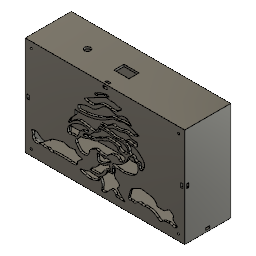
Classroom quality sensor (Autodesk Fusion 360 design; units mm, degrees)
Autodesk Fusion 360 part; units mm, degrees
(part 1 of 2)
sketch "Box (main and holes)" plane through (0, 0, 0) normal (0, 0, 1) x (1, 0, 0)
  line L0 (77.5, 47.5) -> (-77.5, 47.5)
  line L1 (-77.5, 47.5) -> (-77.5, -47.5)
  line L2 (-77.5, -47.5) -> (77.5, -47.5)
  line L3 (77.5, -47.5) -> (77.5, 47.5)
  line L4 (77.5, 47.5) -> (-77.5, -47.5) construction
  line L5 (-77.5, 47.5) -> (77.5, -47.5) construction
  line L6 (-79.5, 49.5) -> (79.5, 49.5)
  line L7 (79.5, 49.5) -> (79.5, -49.5)
  line L8 (79.5, -49.5) -> (-79.5, -49.5)
  line L9 (-79.5, -49.5) -> (-79.5, 49.5)
  line L10 (-79.5, 49.5) -> (79.5, -49.5) construction
  line L11 (79.5, 49.5) -> (-79.5, -49.5) construction
  line L12 (-77.5, -47.5) -> (-77.5, -49.5)
  line L13 (77.5, -47.5) -> (77.5, -49.5)
  dimension "d5" = 155
  dimension "d6" = 95
  dimension "d7" = 2
  dimension "d8" = 2
  constraint horizontal L0
  constraint perpendicular L0 L1
  constraint parallel L0 L2
  constraint parallel L1 L3
  constraint coincident L4 origin
  constraint coincident L5 origin
  constraint horizontal L6
  constraint perpendicular L6 L7
  constraint parallel L6 L8
  constraint parallel L7 L9
  constraint coincident L10 origin
  constraint coincident L11 origin
  constraint coincident L8 L12.end
  constraint perpendicular L8 L12
  constraint coincident L8 L13.end
  constraint perpendicular L8 L13
  measures "d5" distance of L1.end L2.end
  measures "d6" distance of L0.end L1.end
  measures "d7" distance of L2 L8
  measures "d8" distance of L1 L9
extrude "Extrude1" add sketch "Box (main and holes)" against normal blind 2 makes body 1
extrude "Extrude2" add sketch "Box (main and holes)" along normal blind 44 contours L0 L1 L3 L6 L7 L8 L9 L12 L13 bodies 1
chamfer "Chamfer2" distance 2 angle 45 6 edges at (0, -49.5, 0) (-77.5, -49.5, 22) (-77.5, -1, 44) (77.5, -49.5, 22) (77.5, -1, 44) (0, 47.5, 44) on bodies 1
sketch "Box (guides and top holes)" plane through (0, 47.5, 0) normal (0, -1, 0) x (1, 0, 0)
  line L0 (77.5, 42) -> (-77.5, 42)
  line L1 (-77.5, 42) -> (-77.5, 0)
  line L2 (-77.5, 0) -> (77.5, 0)
  line L3 (77.5, 0) -> (77.5, 42)
  line L4 (-77.5, 5) -> (-72.5, 5)
  line L5 (-72.5, 5) -> (-72.5, 7)
  line L6 (-72.5, 7) -> (-77.5, 7)
  line L7 (-77.5, 7) -> (-77.5, 5)
  line L8 (-77.5, 10) -> (-72.5, 10)
  line L9 (-72.5, 10) -> (-72.5, 12)
  line L10 (-72.5, 12) -> (-77.5, 12)
  line L11 (-77.5, 12) -> (-77.5, 10)
  line L12 (-77.5, 42) -> (77.5, 42) construction
  line L13 (72.5, 12) -> (77.5, 12)
  line L14 (77.5, 12) -> (77.5, 10)
  line L15 (77.5, 10) -> (72.5, 10)
  line L16 (72.5, 10) -> (72.5, 12)
  line L17 (72.5, 7) -> (77.5, 7)
  line L18 (77.5, 7) -> (77.5, 5)
  line L19 (77.5, 5) -> (72.5, 5)
  line L20 (72.5, 5) -> (72.5, 7)
  line L21 (0, 1.75) -> (0, 22.5)
  line L22 (2, 42) -> (-2, 42)
  line L23 (-2, 42) -> (-2, 40)
  line L24 (-2, 40) -> (2, 40)
  line L25 (2, 40) -> (2, 42)
  line L26 (2, 42) -> (-2, 40) construction
  line L27 (-2, 42) -> (2, 40) construction
  line L28 (-77.5, 10) -> (77.5, 10) construction
  line L29 (0, 10) -> (0, 22.5) construction
  line L30 (7.5, 27.5) -> (-7.5, 27.5)
  line L31 (-7.5, 27.5) -> (-7.5, 17.5)
  line L32 (-7.5, 17.5) -> (7.5, 17.5)
  line L33 (7.5, 17.5) -> (7.5, 27.5)
  line L34 (7.5, 27.5) -> (-7.5, 17.5) construction
  line L35 (-7.5, 27.5) -> (7.5, 17.5) construction
  line L36 (-38.75, 10) -> (-38.75, 22.5) construction
  circle A0 centre (-38.75, 22.5) radius 3
  point P0 (0, 41)
  point P1 (0, 42)
  point P2 (0, 42)
  point P3 (0, 22.5)
  dimension "d15" = 5
  dimension "d16" = 2
  dimension "d23" = 5
  dimension "d26" = 3
  dimension "d27" = 30
  dimension "d31" = 4
  dimension "d32" = 2
  dimension "d51" = 12.5
  dimension "d52" = 15
  dimension "d53" = 10
  dimension "d54" = 12.5
  dimension "d55" = 38.75
  dimension "d56" = 6
  constraint horizontal L4
  constraint vertical L5
  constraint horizontal L6
  constraint vertical L7
  constraint coincident L1 L4.start
  constraint horizontal L8
  constraint vertical L9
  constraint horizontal L10
  constraint vertical L11
  constraint coincident L1 L8.start
  constraint coincident L1 L0.end
  constraint coincident L3 L0.start
  constraint perpendicular L3 L12
  constraint equal L6 L10
  constraint equal L5 L9
  constraint horizontal L13
  constraint vertical L14
  constraint horizontal L15
  constraint vertical L16
  constraint horizontal L17
  constraint vertical L18
  constraint horizontal L19
  constraint vertical L20
  constraint symmetric L9 L16 L21
  constraint symmetric L8 L15 L21
  constraint symmetric L10 L13 L21
  constraint symmetric L11 L14 L21
  constraint symmetric L4 L19 L21
  constraint symmetric L6 L17 L21
  constraint symmetric L7 L18 L21
  constraint symmetric L5 L20 L21
  constraint horizontal L22
  constraint perpendicular L22 L23
  constraint parallel L22 L24
  constraint parallel L23 L25
  constraint coincident L26 P0
  constraint coincident L27 P0
  constraint midpoint L22 P2
  constraint midpoint L0 P2
  constraint coincident P2 P1
  constraint perpendicular L11 L28
  constraint perpendicular L28 L29
  constraint horizontal L30
  constraint perpendicular L30 L31
  constraint parallel L30 L32
  constraint parallel L31 L33
  constraint coincident L34 P3
  constraint coincident L35 P3
  constraint coincident P3 L21.end
  constraint midpoint L28 L29.start
  constraint coincident L14.end L15.start
  constraint coincident L28 L36.start
  constraint perpendicular L28 L36
  constraint coincident L36.end A0.centre
  measures "d15" distance of L4.start L4.end
  measures "d16" distance of L4.start L6.end
  measures "d23" distance of L2 L4
  measures "d26" distance of L6 L8
  measures "d27" distance of L10 L12
  measures "d31" distance of L23.end L24.end
  measures "d32" distance of L22.end L23.end
  measures "d51" distance of L29.start P3
  measures "d52" distance of L31.end L32.end
  measures "d53" distance of L30.end L31.end
  measures "d54" distance of L36.start L36.end
  measures "d55" distance of L29 L36
  measures "d56" diameter of A0
extrude "Extrude8" cut sketch "Box (guides and top holes)" against normal up to surface (2 mm away) contours L30 L31 L32 L33 | A0 bodies 1
extrude "Extrude3" add sketch "Box (guides and top holes)" along normal blind 95 contours L3 L13 L14 L15 L16 | L3 L17 L18 L19 L20 | L1 L8 L9 L10 L11 | L1 L4 L5 L6 L7 bodies 1
extrude "Extrude4" cut sketch "Box (guides and top holes)" against normal up to surface (2 mm away) contours L0 L22 L23 L24 L25 bodies 1
sketch "Box (back hole)" plane through (0, 0, -2) normal (0, 0, -1) x (-1, 0, 0)
  line L0 (-79.5, -49.5) -> (79.5, -49.5)
  line L1 (79.5, -49.5) -> (79.5, 49.5)
  line L2 (79.5, 49.5) -> (-79.5, 49.5)
  line L3 (-79.5, 49.5) -> (-79.5, -49.5)
  line L4 (2, -45.5) -> (-2, -45.5)
  line L5 (-2, -45.5) -> (-2, -47.5)
  line L6 (-2, -47.5) -> (2, -47.5)
  line L7 (2, -47.5) -> (2, -45.5)
  line L8 (2, -45.5) -> (-2, -47.5) construction
  line L9 (-2, -45.5) -> (2, -47.5) construction
  line L10 (0, -49.5) -> (0, -47.5) construction
  point P0 (0, -46.5)
  point P1 (0, -47.5)
  dimension "d36" = 4
  dimension "d37" = 2
  dimension "d48" = 2
  constraint horizontal L4
  constraint perpendicular L4 L5
  constraint parallel L4 L6
  constraint parallel L5 L7
  constraint coincident L8 P0
  constraint coincident L9 P0
  constraint midpoint L6 P1
  constraint midpoint L0 L10.start
  constraint perpendicular L0 L10
  constraint coincident P1 L10.end
  measures "d36" distance of L5.end L6.end
  measures "d37" distance of L4.end L5.end
  measures "d48" distance of L10.start P1
extrude "Extrude7" cut sketch "Box (back hole)" against normal up to surface (2 mm away) contours L4 L5 L6 L7 bodies 1
extrude "Extrude5" cut sketch "Box (back hole)" against normal up to surface (2 mm away) contours L4 L5 L6 L7 bodies 1
sketch "Box (side holes)" plane through (79.5, 0, 0) normal (1, 0, 0) x (0, 0, -1)
  line L0 (-44, -49.5) -> (2, -49.5)
  line L1 (2, -49.5) -> (2, 49.5)
  line L2 (2, 49.5) -> (-44, 49.5)
  line L3 (-44, 49.5) -> (-44, -49.5)
  line L4 (-21, -49.5) -> (-21, -47.5) construction
  line L5 (-44, 0) -> (-42, 0) construction
  line L6 (-42, 2) -> (-40, 2)
  line L7 (-40, 2) -> (-40, -2)
  line L8 (-40, -2) -> (-42, -2)
  line L9 (-42, -2) -> (-42, 2)
  line L10 (-42, 2) -> (-40, -2) construction
  line L11 (-40, 2) -> (-42, -2) construction
  line L12 (-19, -45.5) -> (-23, -45.5)
  line L13 (-23, -45.5) -> (-23, -47.5)
  line L14 (-23, -47.5) -> (-19, -47.5)
  line L15 (-19, -47.5) -> (-19, -45.5)
  line L16 (-19, -45.5) -> (-23, -47.5) construction
  line L17 (-23, -45.5) -> (-19, -47.5) construction
  point P0 (-41, 0)
  point P1 (-21, -46.5)
  point P2 (-42, 0)
  point P3 (-21, -47.5)
  dimension "d40" = 2
  dimension "d41" = 2
  dimension "d42" = 2
  dimension "d43" = 4
  dimension "d44" = 4
  dimension "d45" = 2
  constraint midpoint L0 L4.start
  constraint vertical L4
  constraint midpoint L3 L5.start
  constraint horizontal L5
  constraint horizontal L6
  constraint perpendicular L6 L7
  constraint parallel L6 L8
  constraint parallel L7 L9
  constraint coincident L10 P0
  constraint coincident L11 P0
  constraint horizontal L12
  constraint perpendicular L12 L13
  constraint parallel L12 L14
  constraint parallel L13 L15
  constraint coincident L16 P1
  constraint coincident L17 P1
  constraint midpoint L9 P2
  constraint coincident L5 P2
  constraint coincident P2 L5.end
  constraint midpoint L14 P3
  constraint coincident L4 P3
  constraint coincident P3 L4.end
  measures "d40" distance of L4.start P3
  measures "d41" distance of L5.start P2
  measures "d42" distance of L7.end L8.end
  measures "d43" distance of L6.end L7.end
  measures "d44" distance of L13.end L14.end
  measures "d45" distance of L12.end L13.end
extrude "Extrude6" cut sketch "Box (side holes)" against normal up to surface (159 mm away) contours L6 L7 L8 L9 | L12 L13 L14 L15 bodies 1
ref_plane "WorkPlane4" through (77.5, -2, 42) normal (0, 0, 1) x (1, 0, 0)
sketch "Lid (main and holes)" plane through (77.5, -2, 42) normal (0, 0, 1) x (1, 0, 0)
  line L0 (0, 49.5) -> (-155, 49.5) construction
  line L1 (-155, 49.5) -> (-155, -45.5) construction
  line L2 (-155, -45.5) -> (0, -45.5)
  line L3 (0, -45.5) -> (0, 49.5) construction
  line L4 (0, -45.5) -> (-155, 49.5) construction
  line L5 (0, 49.5) -> (-155, -45.5) construction
  line L6 (2, 51.5) -> (-157, 51.5)
  line L7 (-157, 51.5) -> (-157, -47.5)
  line L8 (-157, -47.5) -> (2, -47.5)
  line L9 (2, -47.5) -> (2, 51.5)
  line L10 (2, 51.5) -> (-157, -47.5) construction
  line L11 (-157, 51.5) -> (2, -47.5) construction
  line L12 (-155, -45.5) -> (-157, -45.5)
  line L13 (0, -45.5) -> (2, -45.5)
  spline S0 degree 3 poles (-80.6772, -42.0006) (-80.6772, -41.7695) (-80.5006, -40.5665) (-80.2848, -39.3272) knots 0 0 0 0 1 1 1 1
  spline S1 degree 3 poles (-80.2848, -39.3272) (-79.814, -36.6234) (-80.4696, -33.7851) (-81.9287, -32.2107) knots 0 0 0 0 1 1 1 1
  spline S2 degree 3 poles (-81.9287, -32.2107) (-82.4275, -31.6725) (-82.8356, -31.1623) (-82.8356, -31.0769) knots 0 0 0 0 1 1 1 1
  spline S3 degree 3 poles (-82.8356, -31.0769) (-82.8356, -30.9915) (-82.0667, -30.5302) (-81.1269, -30.0518) knots 0 0 0 0 1 1 1 1
  spline S4 degree 3 poles (-81.1269, -30.0518) (-79.0239, -28.9814) (-78.0158, -27.9242) (-76.3554, -25.048) knots 0 0 0 0 1 1 1 1
  line L14 (-76.3554, -25.048) -> (-75.0666, -22.8156)
  line L15 (-75.0666, -22.8156) -> (-72.386, -22.6357)
  line L16 (-72.386, -22.6357) -> (-69.7055, -22.4559)
  line L17 (-69.7055, -22.4559) -> (-69.7714, -21.3767)
  spline S5 degree 3 poles (-69.7714, -21.3767) (-69.8076, -20.7831) (-69.9513, -19.4305) (-70.0906, -18.3708) knots 0 0 0 0 1 1 1 1
  spline S6 degree 3 poles (-70.0906, -18.3708) (-70.2833, -16.9057) (-70.2244, -16.3683) (-69.8448, -16.128) knots 0 0 0 0 1 1 1 1
  spline S7 degree 3 poles (-69.8448, -16.128) (-68.9821, -15.5816) (-67.7675, -15.7724) (-67.3691, -16.5169) knots 0 0 0 0 1 1 1 1
  spline S8 degree 3 poles (-67.3691, -16.5169) (-66.7637, -17.6481) (-66.8262, -19.6808) (-67.4889, -20.4131) knots 0 0 0 0 1 1 1 1
  spline S9 degree 3 poles (-67.4889, -20.4131) (-68.1856, -21.1828) (-68.2166, -21.6138) (-67.7076, -23.4466) knots 0 0 0 0 1 1 1 1
  spline S10 degree 3 poles (-67.7076, -23.4466) (-67.4212, -24.4779) (-67.0046, -24.9645) (-65.945, -25.5051) knots 0 0 0 0 1 1 1 1
  spline S11 degree 3 poles (-65.945, -25.5051) (-63.0081, -27.0033) (-62.1719, -29.5189) (-64.1297, -30.9664) knots 0 0 0 0 1 1 1 1
  spline S12 degree 3 poles (-64.1297, -30.9664) (-64.7232, -31.4052) (-65.2089, -31.9006) (-65.2089, -32.0672) knots 0 0 0 0 1 1 1 1
  spline S13 degree 3 poles (-65.2089, -32.0672) (-65.2089, -32.6272) (-61.1292, -37.1914) (-59.3835, -38.5843) knots 0 0 0 0 1 1 1 1
  spline S14 degree 3 poles (-59.3835, -38.5843) (-57.2217, -40.3093) (-57.1711, -40.7788) (-59.1834, -40.4415) knots 0 0 0 0 1 1 1 1
  spline S15 degree 3 poles (-59.1834, -40.4415) (-60.0243, -40.3005) (-61.9999, -40.1621) (-63.5737, -40.1339) knots 0 0 0 0 1 1 1 1
  line L18 (-63.5737, -40.1339) -> (-66.4351, -40.0826)
  line L19 (-66.4351, -40.0826) -> (-66.6875, -38.8568)
  spline S16 degree 3 poles (-66.6875, -38.8568) (-66.9456, -37.6031) (-67.4468, -37.1486) (-69.3475, -36.4447) knots 0 0 0 0 1 1 1 1
  spline S17 degree 3 poles (-69.3475, -36.4447) (-70.9168, -35.8635) (-71.7946, -36.3434) (-73.7366, -38.8441) knots 0 0 0 0 1 1 1 1
  spline S18 degree 3 poles (-73.7366, -38.8441) (-74.681, -40.0602) (-76.0559, -41.3625) (-76.7921, -41.738) knots 0 0 0 0 1 1 1 1
  spline S19 degree 3 poles (-76.7921, -41.738) (-78.2809, -42.4976) (-80.6772, -42.6595) (-80.6772, -42.0006) knots 0 0 0 0 1 1 1 1
  spline S20 degree 3 poles (-24.7596, -37.8921) (-27.8966, -35.337) (-29.9959, -34.4364) (-33.7454, -34.0371) knots 0 0 0 0 1 1 1 1
  spline S21 degree 3 poles (-33.7454, -34.0371) (-36.4215, -33.7522) (-37.1897, -33.7852) (-38.0213, -34.2209) knots 0 0 0 0 1 1 1 1
  spline S22 degree 3 poles (-38.0213, -34.2209) (-38.8905, -34.6763) (-39.3237, -34.684) (-41.0603, -34.2753) knots 0 0 0 0 1 1 1 1
  spline S23 degree 3 poles (-41.0603, -34.2753) (-44.0129, -33.5803) (-44.5843, -33.6582) (-45.6908, -34.9066) knots 0 0 0 0 1 1 1 1
  spline S24 degree 3 poles (-45.6908, -34.9066) (-47.056, -36.447) (-48.0082, -36.751) (-49.5063, -36.1251) knots 0 0 0 0 1 1 1 1
  spline S25 degree 3 poles (-49.5063, -36.1251) (-50.4112, -35.747) (-51.0532, -35.7031) (-51.9439, -35.9586) knots 0 0 0 0 1 1 1 1
  spline S26 degree 3 poles (-51.9439, -35.9586) (-53.6167, -36.4384) (-53.5786, -36.4579) (-53.8158, -34.9965) knots 0 0 0 0 1 1 1 1
  spline S27 degree 3 poles (-53.8158, -34.9965) (-53.9563, -34.1306) (-53.8505, -33.4339) (-53.5031, -32.938) knots 0 0 0 0 1 1 1 1
  spline S28 degree 3 poles (-53.5031, -32.938) (-53.2143, -32.5257) (-52.9781, -31.5491) (-52.9781, -30.7678) knots 0 0 0 0 1 1 1 1
  spline S29 degree 3 poles (-52.9781, -30.7678) (-52.9781, -29.964) (-52.7254, -29.0682) (-52.396, -28.7042) knots 0 0 0 0 1 1 1 1
  spline S30 degree 3 poles (-52.396, -28.7042) (-52.0759, -28.3505) (-51.7066, -27.5284) (-51.5753, -26.8773) knots 0 0 0 0 1 1 1 1
  spline S31 degree 3 poles (-51.5753, -26.8773) (-51.3335, -25.6784) (-50.0936, -24.7772) (-46.5029, -23.1905) knots 0 0 0 0 1 1 1 1
  spline S32 degree 3 poles (-46.5029, -23.1905) (-45.8105, -22.8845) (-44.4126, -22.2051) (-43.3967, -21.6807) knots 0 0 0 0 1 1 1 1
  spline S33 degree 3 poles (-43.3967, -21.6807) (-41.6649, -20.7868) (-41.4176, -20.7518) (-39.4397, -21.1199) knots 0 0 0 0 1 1 1 1
  spline S34 degree 3 poles (-39.4397, -21.1199) (-38.2793, -21.3359) (-35.792, -21.7073) (-33.9124, -21.9454) knots 0 0 0 0 1 1 1 1
  spline S35 degree 3 poles (-33.9124, -21.9454) (-30.1865, -22.4172) (-29.7107, -22.5865) (-27.7144, -24.1512) knots 0 0 0 0 1 1 1 1
  spline S36 degree 3 poles (-27.7144, -24.1512) (-26.8336, -24.8415) (-26.2438, -25.6812) (-25.9976, -26.5955) knots 0 0 0 0 1 1 1 1
  spline S37 degree 3 poles (-25.9976, -26.5955) (-25.5767, -28.1587) (-25.2264, -28.3349) (-22.4011, -28.4042) knots 0 0 0 0 1 1 1 1
  spline S38 degree 3 poles (-22.4011, -28.4042) (-18.1103, -28.5095) (-17.9926, -28.4793) (-16.0416, -26.7726) knots 0 0 0 0 1 1 1 1
  spline S39 degree 3 poles (-16.0416, -26.7726) (-13.6839, -24.7101) (-12.8952, -24.7039) (-10.6571, -26.7302) knots 0 0 0 0 1 1 1 1
  spline S40 degree 3 poles (-10.6571, -26.7302) (-8.9354, -28.289) (-8.9209, -28.3205) (-9.3632, -29.5437) knots 0 0 0 0 1 1 1 1
  spline S41 degree 3 poles (-9.3632, -29.5437) (-9.6093, -30.224) (-9.8106, -31.0277) (-9.8106, -31.3297) knots 0 0 0 0 1 1 1 1
  spline S42 degree 3 poles (-9.8106, -31.3297) (-9.8106, -31.8271) (-6.9005, -34.6147) (-5.6186, -35.3452) knots 0 0 0 0 1 1 1 1
  spline S43 degree 3 poles (-5.6186, -35.3452) (-4.9673, -35.7164) (-5.4176, -36.3371) (-7.0868, -37.3687) knots 0 0 0 0 1 1 1 1
  line L20 (-7.0868, -37.3687) -> (-8.2392, -38.0809)
  line L21 (-8.2392, -38.0809) -> (-10.6789, -37.2284)
  spline S44 degree 3 poles (-10.6789, -37.2284) (-12.5663, -36.5689) (-13.3748, -36.4493) (-14.2501, -36.7004) knots 0 0 0 0 1 1 1 1
  spline S45 degree 3 poles (-14.2501, -36.7004) (-14.8724, -36.8789) (-15.9978, -37.0249) (-16.7508, -37.0249) knots 0 0 0 0 1 1 1 1
  spline S46 degree 3 poles (-16.7508, -37.0249) (-18.2007, -37.0249) (-19.8766, -37.735) (-21.0861, -38.8618) knots 0 0 0 0 1 1 1 1
  spline S47 degree 3 poles (-21.0861, -38.8618) (-22.1303, -39.8346) (-22.4921, -39.7391) (-24.7596, -37.8921) knots 0 0 0 0 1 1 1 1
  spline S48 degree 3 poles (-97.0237, -36.8253) (-99.636, -36.2564) (-101.2039, -35.7237) (-101.6862, -35.2414) knots 0 0 0 0 1 1 1 1
  spline S49 degree 3 poles (-101.6862, -35.2414) (-102.6768, -34.2508) (-102.2117, -33.9057) (-99.2493, -33.4338) knots 0 0 0 0 1 1 1 1
  spline S50 degree 3 poles (-99.2493, -33.4338) (-97.8896, -33.2172) (-95.8002, -32.6288) (-94.606, -32.1262) knots 0 0 0 0 1 1 1 1
  spline S51 degree 3 poles (-94.606, -32.1262) (-92.6531, -31.3042) (-92.2711, -31.2536) (-90.8061, -31.6225) knots 0 0 0 0 1 1 1 1
  spline S52 degree 3 poles (-90.8061, -31.6225) (-89.9103, -31.8481) (-88.0657, -31.9966) (-86.707, -31.9525) knots 0 0 0 0 1 1 1 1
  spline S53 degree 3 poles (-86.707, -31.9525) (-84.027, -31.8656) (-83.4178, -32.1725) (-83.0166, -33.8116) knots 0 0 0 0 1 1 1 1
  spline S54 degree 3 poles (-83.0166, -33.8116) (-82.8044, -34.6785) (-82.947, -34.7965) (-85.3372, -35.7343) knots 0 0 0 0 1 1 1 1
  spline S55 degree 3 poles (-85.3372, -35.7343) (-88.2851, -36.8909) (-91.3347, -37.7474) (-92.3684, -37.7092) knots 0 0 0 0 1 1 1 1
  spline S56 degree 3 poles (-92.3684, -37.7092) (-92.7641, -37.6945) (-94.859, -37.2968) (-97.0237, -36.8253) knots 0 0 0 0 1 1 1 1
  spline S57 degree 3 poles (-147.6773, -33.1249) (-149.078, -32.2806) (-149.8129, -30.56) (-149.5295, -28.788) knots 0 0 0 0 1 1 1 1
  spline S58 degree 3 poles (-149.5295, -28.788) (-149.2574, -27.0861) (-149.5277, -25.7824) (-150.3164, -24.9937) knots 0 0 0 0 1 1 1 1
  spline S59 degree 3 poles (-150.3164, -24.9937) (-150.8367, -24.4734) (-150.7749, -24.377) (-149.608, -23.8894) knots 0 0 0 0 1 1 1 1
  spline S60 degree 3 poles (-149.608, -23.8894) (-148.9047, -23.5956) (-147.5975, -23.3552) (-146.7029, -23.3552) knots 0 0 0 0 1 1 1 1
  spline S61 degree 3 poles (-146.7029, -23.3552) (-145.2585, -23.3552) (-144.8568, -23.554) (-143.1154, -25.131) knots 0 0 0 0 1 1 1 1
  spline S62 degree 3 poles (-143.1154, -25.131) (-141.2401, -26.8293) (-139.4115, -27.6656) (-137.5638, -27.6699) knots 0 0 0 0 1 1 1 1
  spline S63 degree 3 poles (-137.5638, -27.6699) (-136.7109, -27.6721) (-135.9042, -27.1103) (-132.3442, -24.0357) knots 0 0 0 0 1 1 1 1
  spline S64 degree 3 poles (-132.3442, -24.0357) (-130.4413, -22.3922) (-128.5635, -21.616) (-123.6648, -20.4479) knots 0 0 0 0 1 1 1 1
  spline S65 degree 3 poles (-123.6648, -20.4479) (-122.6756, -20.212) (-121.08, -19.811) (-120.1192, -19.5569) knots 0 0 0 0 1 1 1 1
  spline S66 degree 3 poles (-120.1192, -19.5569) (-118.5035, -19.1295) (-118.1725, -19.1652) (-115.7156, -20.0312) knots 0 0 0 0 1 1 1 1
  spline S67 degree 3 poles (-115.7156, -20.0312) (-113.1416, -20.9386) (-112.9692, -20.9531) (-110.1634, -20.4975) knots 0 0 0 0 1 1 1 1
  spline S68 degree 3 poles (-110.1634, -20.4975) (-108.5707, -20.2388) (-107.2219, -20.088) (-107.1659, -20.1624) knots 0 0 0 0 1 1 1 1
  spline S69 degree 3 poles (-107.1659, -20.1624) (-107.11, -20.2367) (-106.6991, -20.826) (-106.253, -21.472) knots 0 0 0 0 1 1 1 1
  spline S70 degree 3 poles (-106.253, -21.472) (-105.2416, -22.9364) (-104.0504, -23.5587) (-101.6314, -23.8864) knots 0 0 0 0 1 1 1 1
  spline S71 degree 3 poles (-101.6314, -23.8864) (-100.5927, -24.027) (-99.7429, -24.2704) (-99.7429, -24.4272) knots 0 0 0 0 1 1 1 1
  spline S72 degree 3 poles (-99.7429, -24.4272) (-99.7429, -24.5839) (-100.6996, -25.4126) (-101.869, -26.2687) knots 0 0 0 0 1 1 1 1
  spline S73 degree 3 poles (-101.869, -26.2687) (-104.3873, -28.1125) (-105.2183, -29.3428) (-104.9275, -30.7969) knots 0 0 0 0 1 1 1 1
  spline S74 degree 3 poles (-104.9275, -30.7969) (-104.7346, -31.7612) (-104.8516, -31.8997) (-106.5191, -32.6807) knots 0 0 0 0 1 1 1 1
  spline S75 degree 3 poles (-106.5191, -32.6807) (-108.2756, -33.5034) (-108.4039, -33.5123) (-111.855, -33.052) knots 0 0 0 0 1 1 1 1
  spline S76 degree 3 poles (-111.855, -33.052) (-116.5865, -32.4208) (-127.3185, -32.5432) (-129.3514, -33.2515) knots 0 0 0 0 1 1 1 1
  spline S77 degree 3 poles (-129.3514, -33.2515) (-131.3613, -33.9517) (-131.7467, -33.924) (-132.7202, -33.0095) knots 0 0 0 0 1 1 1 1
  spline S78 degree 3 poles (-132.7202, -33.0095) (-133.4658, -32.3091) (-133.6868, -32.2733) (-134.9435, -32.6498) knots 0 0 0 0 1 1 1 1
  spline S79 degree 3 poles (-134.9435, -32.6498) (-136.7787, -33.1997) (-138.2081, -33.1599) (-139.3131, -32.5283) knots 0 0 0 0 1 1 1 1
  spline S80 degree 3 poles (-139.3131, -32.5283) (-140.6294, -31.7758) (-141.7024, -31.8753) (-143.1928, -32.888) knots 0 0 0 0 1 1 1 1
  spline S81 degree 3 poles (-143.1928, -32.888) (-144.7042, -33.915) (-146.2326, -33.9957) (-147.6773, -33.1249) knots 0 0 0 0 1 1 1 1
  spline S82 degree 3 poles (-91.559, -29.5823) (-92.208, -29.4128) (-92.4461, -28.7511) (-91.8582, -28.7511) knots 0 0 0 0 1 1 1 1
  spline S83 degree 3 poles (-91.8582, -28.7511) (-91.6764, -28.7511) (-91.188, -28.2014) (-90.7728, -27.5295) knots 0 0 0 0 1 1 1 1
  spline S84 degree 3 poles (-90.7728, -27.5295) (-90.3338, -26.8192) (-89.6063, -26.2078) (-89.0347, -26.0687) knots 0 0 0 0 1 1 1 1
  spline S85 degree 3 poles (-89.0347, -26.0687) (-87.209, -25.6244) (-85.3185, -24.0865) (-84.5991, -22.4602) knots 0 0 0 0 1 1 1 1
  spline S86 degree 3 poles (-84.5991, -22.4602) (-83.7854, -20.6207) (-81.6889, -19.3982) (-79.3479, -19.3982) knots 0 0 0 0 1 1 1 1
  spline S87 degree 3 poles (-79.3479, -19.3982) (-78.1639, -19.3982) (-77.4896, -19.0904) (-75.8013, -17.7794) knots 0 0 0 0 1 1 1 1
  spline S88 degree 3 poles (-75.8013, -17.7794) (-74.6547, -16.889) (-73.5945, -16.1606) (-73.4453, -16.1606) knots 0 0 0 0 1 1 1 1
  spline S89 degree 3 poles (-73.4453, -16.1606) (-73.2961, -16.1606) (-72.9175, -17.0427) (-72.6041, -18.1208) knots 0 0 0 0 1 1 1 1
  spline S90 degree 3 poles (-72.6041, -18.1208) (-72.2907, -19.1989) (-71.8745, -20.1797) (-71.6793, -20.3004) knots 0 0 0 0 1 1 1 1
  spline S91 degree 3 poles (-71.6793, -20.3004) (-71.484, -20.4211) (-71.3243, -20.7354) (-71.3243, -20.9989) knots 0 0 0 0 1 1 1 1
  spline S92 degree 3 poles (-71.3243, -20.9989) (-71.3243, -21.3426) (-72.0775, -21.5159) (-73.9904, -21.6125) knots 0 0 0 0 1 1 1 1
  spline S93 degree 3 poles (-73.9904, -21.6125) (-77.0757, -21.7683) (-77.5848, -22.0995) (-79.2355, -25.0243) knots 0 0 0 0 1 1 1 1
  spline S94 degree 3 poles (-79.2355, -25.0243) (-80.483, -27.2348) (-82.0314, -28.745) (-83.6738, -29.3533) knots 0 0 0 0 1 1 1 1
  spline S95 degree 3 poles (-83.6738, -29.3533) (-84.773, -29.7603) (-90.2671, -29.9199) (-91.559, -29.5823) knots 0 0 0 0 1 1 1 1
  spline S96 degree 3 poles (-101.7214, -19.0971) (-103.2096, -18.1895) (-104.9681, -16.1138) (-106.0388, -14.0009) knots 0 0 0 0 1 1 1 1
  spline S97 degree 3 poles (-106.0388, -14.0009) (-107.3671, -11.3796) (-107.2513, -10.7008) (-105.3152, -9.7601) knots 0 0 0 0 1 1 1 1
  spline S98 degree 3 poles (-105.3152, -9.7601) (-103.9345, -9.0894) (-102.6025, -7.6309) (-102.152, -6.2967) knots 0 0 0 0 1 1 1 1
  spline S99 degree 3 poles (-102.152, -6.2967) (-102.0905, -6.1145) (-100.8643, -5.8399) (-99.427, -5.6863) knots 0 0 0 0 1 1 1 1
  spline S100 degree 3 poles (-99.427, -5.6863) (-97.6101, -5.4922) (-96.3089, -5.1112) (-95.1568, -4.436) knots 0 0 0 0 1 1 1 1
  spline S101 degree 3 poles (-95.1568, -4.436) (-93.9226, -3.7127) (-92.8505, -3.42) (-90.9555, -3.2891) knots 0 0 0 0 1 1 1 1
  spline S102 degree 3 poles (-90.9555, -3.2891) (-88.1673, -3.0964) (-84.0692, -1.368) (-83.0917, 0.0275) knots 0 0 0 0 1 1 1 1
  spline S103 degree 3 poles (-83.0917, 0.0275) (-82.7663, 0.4921) (-81.5918, 1.0352) (-79.9175, 1.4953) knots 0 0 0 0 1 1 1 1
  spline S104 degree 3 poles (-79.9175, 1.4953) (-78.4558, 1.8969) (-76.6359, 2.6347) (-75.8734, 3.1347) knots 0 0 0 0 1 1 1 1
  spline S105 degree 3 poles (-75.8734, 3.1347) (-74.1779, 4.2467) (-71.5713, 4.5654) (-68.6263, 4.0208) knots 0 0 0 0 1 1 1 1
  spline S106 degree 3 poles (-68.6263, 4.0208) (-66.174, 3.5673) (-64.7796, 2.6967) (-64.4826, 1.4337) knots 0 0 0 0 1 1 1 1
  spline S107 degree 3 poles (-64.4826, 1.4337) (-64.3176, 0.7322) (-63.637, 0.311) (-60.9147, -0.7741) knots 0 0 0 0 1 1 1 1
  spline S108 degree 3 poles (-60.9147, -0.7741) (-59.0645, -1.5117) (-57.4714, -2.1945) (-57.3744, -2.2915) knots 0 0 0 0 1 1 1 1
  spline S109 degree 3 poles (-57.3744, -2.2915) (-57.2774, -2.3885) (-57.3685, -2.9182) (-57.5769, -3.4686) knots 0 0 0 0 1 1 1 1
  spline S110 degree 3 poles (-57.5769, -3.4686) (-57.7853, -4.0191) (-58.0525, -4.9125) (-58.1706, -5.4541) knots 0 0 0 0 1 1 1 1
  spline S111 degree 3 poles (-58.1706, -5.4541) (-58.4333, -6.6581) (-59.5265, -7.417) (-61.4317, -7.7182) knots 0 0 0 0 1 1 1 1
  spline S112 degree 3 poles (-61.4317, -7.7182) (-62.7564, -7.9275) (-62.921, -7.8597) (-63.505, -6.8633) knots 0 0 0 0 1 1 1 1
  spline S113 degree 3 poles (-63.505, -6.8633) (-64.3704, -5.3867) (-66.0662, -4.8645) (-68.5176, -5.3199) knots 0 0 0 0 1 1 1 1
  spline S114 degree 3 poles (-68.5176, -5.3199) (-71.3848, -5.8524) (-72.0781, -6.2126) (-73.8133, -8.0707) knots 0 0 0 0 1 1 1 1
  spline S115 degree 3 poles (-73.8133, -8.0707) (-76.5151, -10.9639) (-78.2988, -11.3147) (-83.445, -9.965) knots 0 0 0 0 1 1 1 1
  line L22 (-83.445, -9.965) -> (-86.4941, -9.1653)
  line L23 (-86.4941, -9.1653) -> (-89.0715, -10.5562)
  spline S116 degree 3 poles (-89.0715, -10.5562) (-92.5993, -12.4601) (-92.908, -12.7746) (-92.908, -14.4652) knots 0 0 0 0 1 1 1 1
  spline S117 degree 3 poles (-92.908, -14.4652) (-92.908, -16.1151) (-93.928, -17.9717) (-95.4171, -19.032) knots 0 0 0 0 1 1 1 1
  spline S118 degree 3 poles (-95.4171, -19.032) (-96.7747, -19.9987) (-100.1852, -20.0339) (-101.7214, -19.0971) knots 0 0 0 0 1 1 1 1
  spline S119 degree 3 poles (-84.1836, -18.7518) (-84.4559, -18.5732) (-84.7245, -17.1579) (-84.867, -15.1507) knots 0 0 0 0 1 1 1 1
  line L24 (-84.867, -15.1507) -> (-85.1017, -11.8438)
  line L25 (-85.1017, -11.8438) -> (-82.6905, -11.8438)
  spline S120 degree 3 poles (-82.6905, -11.8438) (-80.7229, -11.8438) (-80.0402, -12.0064) (-78.9793, -12.7273) knots 0 0 0 0 1 1 1 1
  spline S121 degree 3 poles (-78.9793, -12.7273) (-77.6504, -13.6302) (-77.0799, -13.6324) (-77.0799, -12.7346) knots 0 0 0 0 1 1 1 1
  spline S122 degree 3 poles (-77.0799, -12.7346) (-77.0799, -11.9031) (-75.9431, -11.564) (-73.7834, -11.7512) knots 0 0 0 0 1 1 1 1
  spline S123 degree 3 poles (-73.7834, -11.7512) (-72.2283, -11.886) (-71.7065, -12.0788) (-71.5792, -12.5655) knots 0 0 0 0 1 1 1 1
  spline S124 degree 3 poles (-71.5792, -12.5655) (-71.3205, -13.5547) (-71.7828, -13.9941) (-73.6847, -14.5665) knots 0 0 0 0 1 1 1 1
  spline S125 degree 3 poles (-73.6847, -14.5665) (-74.6506, -14.8572) (-75.9311, -15.5693) (-76.5302, -16.149) knots 0 0 0 0 1 1 1 1
  spline S126 degree 3 poles (-76.5302, -16.149) (-78.3703, -17.9294) (-83.0242, -19.5121) (-84.1836, -18.7518) knots 0 0 0 0 1 1 1 1
  spline S127 degree 3 poles (-63.5901, -15.3575) (-67.6701, -14.9857) (-69.6501, -14.4185) (-69.8126, -13.5749) knots 0 0 0 0 1 1 1 1
  spline S128 degree 3 poles (-69.8126, -13.5749) (-69.8988, -13.1273) (-69.5016, -12.9378) (-68.0635, -12.74) knots 0 0 0 0 1 1 1 1
  spline S129 degree 3 poles (-68.0635, -12.74) (-65.0176, -12.3211) (-60.2319, -9.6946) (-57.874, -7.1478) knots 0 0 0 0 1 1 1 1
  spline S130 degree 3 poles (-57.874, -7.1478) (-56.7666, -5.9517) (-55.7546, -4.536) (-55.6249, -4.0018) knots 0 0 0 0 1 1 1 1
  spline S131 degree 3 poles (-55.6249, -4.0018) (-55.2097, -2.2903) (-53.6926, 0.9119) (-53.077, 1.3762) knots 0 0 0 0 1 1 1 1
  spline S132 degree 3 poles (-53.077, 1.3762) (-52.4567, 1.8441) (-49.8593, 1.9869) (-48.8706, 1.6075) knots 0 0 0 0 1 1 1 1
  spline S133 degree 3 poles (-48.8706, 1.6075) (-48.5577, 1.4874) (-48.3016, 1.0216) (-48.3016, 0.5724) knots 0 0 0 0 1 1 1 1
  spline S134 degree 3 poles (-48.3016, 0.5724) (-48.3016, -0.3934) (-47.768, -0.9013) (-46.3904, -1.2471) knots 0 0 0 0 1 1 1 1
  spline S135 degree 3 poles (-46.3904, -1.2471) (-44.8084, -1.6442) (-44.3756, -2.6646) (-44.5346, -5.623) knots 0 0 0 0 1 1 1 1
  spline S136 degree 3 poles (-44.5346, -5.623) (-44.7549, -9.7232) (-46.0501, -11.6202) (-49.9746, -13.5905) knots 0 0 0 0 1 1 1 1
  spline S137 degree 3 poles (-49.9746, -13.5905) (-51.6142, -14.4137) (-57.6231, -15.8348) (-59.0766, -15.7431) knots 0 0 0 0 1 1 1 1
  spline S138 degree 3 poles (-59.0766, -15.7431) (-59.5805, -15.7113) (-61.6116, -15.5378) (-63.5901, -15.3575) knots 0 0 0 0 1 1 1 1
  spline S139 degree 3 poles (-114.2862, -8.7605) (-115.285, -7.7617) (-115.02, -5.027) (-113.7366, -3.0895) knots 0 0 0 0 1 1 1 1
  spline S140 degree 3 poles (-113.7366, -3.0895) (-110.0391, 2.4927) (-101.1224, 6.2764) (-95.9962, 4.4384) knots 0 0 0 0 1 1 1 1
  spline S141 degree 3 poles (-95.9962, 4.4384) (-93.7835, 3.645) (-93.2235, 2.8684) (-94.1366, 1.8596) knots 0 0 0 0 1 1 1 1
  spline S142 degree 3 poles (-94.1366, 1.8596) (-94.804, 1.122) (-97.9387, 0.0272) (-99.383, 0.0272) knots 0 0 0 0 1 1 1 1
  spline S143 degree 3 poles (-99.383, 0.0272) (-101.2669, 0.0272) (-102.9192, -2.024) (-104.2068, -5.9614) knots 0 0 0 0 1 1 1 1
  spline S144 degree 3 poles (-104.2068, -5.9614) (-104.9541, -8.2464) (-106.235, -9.0474) (-108.3735, -8.5669) knots 0 0 0 0 1 1 1 1
  spline S145 degree 3 poles (-108.3735, -8.5669) (-109.3311, -8.3517) (-110.2676, -8.4184) (-111.4878, -8.7886) knots 0 0 0 0 1 1 1 1
  spline S146 degree 3 poles (-111.4878, -8.7886) (-113.6514, -9.445) (-113.6012, -9.4455) (-114.2862, -8.7605) knots 0 0 0 0 1 1 1 1
  spline S147 degree 3 poles (-42.8414, -4.9066) (-43.0523, -4.6525) (-43.2745, -3.4788) (-43.3351, -2.2986) knots 0 0 0 0 1 1 1 1
  line L26 (-43.3351, -2.2986) -> (-43.4453, -0.1527)
  line L27 (-43.4453, -0.1527) -> (-45.4915, -0.0454)
  spline S148 degree 3 poles (-45.4915, -0.0454) (-47.473, 0.0584) (-47.5508, 0.1012) (-47.9485, 1.3063) knots 0 0 0 0 1 1 1 1
  spline S149 degree 3 poles (-47.9485, 1.3063) (-48.4556, 2.843) (-49.37, 3.3669) (-51.0086, 3.0595) knots 0 0 0 0 1 1 1 1
  spline S150 degree 3 poles (-51.0086, 3.0595) (-52.7144, 2.7395) (-53.3378, 3.3295) (-53.3378, 5.2639) knots 0 0 0 0 1 1 1 1
  spline S151 degree 3 poles (-53.3378, 5.2639) (-53.3378, 7.5028) (-53.869, 8.5826) (-55.3082, 9.2689) knots 0 0 0 0 1 1 1 1
  spline S152 degree 3 poles (-55.3082, 9.2689) (-56.3032, 9.7433) (-56.5754, 10.0851) (-56.5754, 10.86) knots 0 0 0 0 1 1 1 1
  spline S153 degree 3 poles (-56.5754, 10.86) (-56.5754, 11.4028) (-56.3233, 12.0989) (-56.0152, 12.407) knots 0 0 0 0 1 1 1 1
  spline S154 degree 3 poles (-56.0152, 12.407) (-55.528, 12.8943) (-55.3525, 12.9012) (-54.6663, 12.4603) knots 0 0 0 0 1 1 1 1
  spline S155 degree 3 poles (-54.6663, 12.4603) (-53.773, 11.8864) (-50.2611, 11.1788) (-48.306, 11.1788) knots 0 0 0 0 1 1 1 1
  spline S156 degree 3 poles (-48.306, 11.1788) (-46.6141, 11.1788) (-44.5032, 9.8193) (-41.268, 6.6461) knots 0 0 0 0 1 1 1 1
  spline S157 degree 3 poles (-41.268, 6.6461) (-38.2459, 3.6819) (-37.5241, 1.9272) (-38.2369, -0.7223) knots 0 0 0 0 1 1 1 1
  spline S158 degree 3 poles (-38.2369, -0.7223) (-39.0522, -3.7526) (-40.2318, -5.3687) (-41.6283, -5.3687) knots 0 0 0 0 1 1 1 1
  spline S159 degree 3 poles (-41.6283, -5.3687) (-42.0845, -5.3687) (-42.6304, -5.1608) (-42.8414, -4.9066) knots 0 0 0 0 1 1 1 1
  spline S160 degree 3 poles (-98.9956, -3.4237) (-99.8234, -2.4262) (-99.1463, -1.8717) (-95.6975, -0.7227) knots 0 0 0 0 1 1 1 1
  spline S161 degree 3 poles (-95.6975, -0.7227) (-92.6011, 0.3088) (-92.1494, 0.583) (-90.2761, 2.568) knots 0 0 0 0 1 1 1 1
  spline S162 degree 3 poles (-90.2761, 2.568) (-88.8264, 4.104) (-87.5527, 5.0383) (-85.8938, 5.7827) knots 0 0 0 0 1 1 1 1
  line L28 (-85.8938, 5.7827) -> (-83.5551, 6.832)
  line L29 (-83.5551, 6.832) -> (-83.5551, 8.4531)
  spline S163 degree 3 poles (-83.5551, 8.4531) (-83.5551, 10.7372) (-83.0724, 10.9148) (-77.274, 10.7635) knots 0 0 0 0 1 1 1 1
  spline S164 degree 3 poles (-77.274, 10.7635) (-73.7134, 10.6705) (-72.3491, 10.5032) (-71.8631, 10.0996) knots 0 0 0 0 1 1 1 1
  spline S165 degree 3 poles (-71.8631, 10.0996) (-71.3448, 9.6692) (-70.0413, 9.56) (-65.4232, 9.56) knots 0 0 0 0 1 1 1 1
  spline S166 degree 3 poles (-65.4232, 9.56) (-59.8581, 9.56) (-59.5561, 9.5222) (-57.6517, 8.5869) knots 0 0 0 0 1 1 1 1
  spline S167 degree 3 poles (-57.6517, 8.5869) (-56.4881, 8.0155) (-55.4117, 7.176) (-55.0437, 6.5529) knots 0 0 0 0 1 1 1 1
  spline S168 degree 3 poles (-55.0437, 6.5529) (-54.1713, 5.0761) (-54.2331, 3.0889) (-55.1809, 2.1411) knots 0 0 0 0 1 1 1 1
  spline S169 degree 3 poles (-55.1809, 2.1411) (-55.8577, 1.4643) (-56.2448, 1.3965) (-58.5769, 1.5461) knots 0 0 0 0 1 1 1 1
  spline S170 degree 3 poles (-58.5769, 1.5461) (-61.6166, 1.7412) (-62.9764, 2.4447) (-63.2837, 3.981) knots 0 0 0 0 1 1 1 1
  spline S171 degree 3 poles (-63.2837, 3.981) (-63.5126, 5.1259) (-63.6374, 5.1742) (-67.9068, 5.7744) knots 0 0 0 0 1 1 1 1
  spline S172 degree 3 poles (-67.9068, 5.7744) (-71.7584, 6.3158) (-75.1438, 6.2305) (-76.4683, 5.5586) knots 0 0 0 0 1 1 1 1
  spline S173 degree 3 poles (-76.4683, 5.5586) (-77.1015, 5.2374) (-78.3935, 4.4246) (-79.3395, 3.7524) knots 0 0 0 0 1 1 1 1
  spline S174 degree 3 poles (-79.3395, 3.7524) (-80.2855, 3.0803) (-81.9486, 2.2987) (-83.0353, 2.0157) knots 0 0 0 0 1 1 1 1
  spline S175 degree 3 poles (-83.0353, 2.0157) (-84.3934, 1.6619) (-85.2941, 1.1646) (-85.9167, 0.4247) knots 0 0 0 0 1 1 1 1
  spline S176 degree 3 poles (-85.9167, 0.4247) (-86.9139, -0.7604) (-90.1095, -2.1244) (-91.9322, -2.1429) knots 0 0 0 0 1 1 1 1
  spline S177 degree 3 poles (-91.9322, -2.1429) (-92.5678, -2.1493) (-93.9782, -2.4834) (-95.0664, -2.8852) knots 0 0 0 0 1 1 1 1
  spline S178 degree 3 poles (-95.0664, -2.8852) (-98.0449, -3.9849) (-98.4803, -4.0446) (-98.9956, -3.4237) knots 0 0 0 0 1 1 1 1
  spline S179 degree 3 poles (-113.7723, 0.5747) (-113.7723, 0.678) (-113.2958, 1.8133) (-112.7135, 3.0976) knots 0 0 0 0 1 1 1 1
  spline S180 degree 3 poles (-112.7135, 3.0976) (-111.973, 4.7308) (-110.9998, 6.0559) (-109.4759, 7.506) knots 0 0 0 0 1 1 1 1
  line L30 (-109.4759, 7.506) -> (-107.2972, 9.5792)
  line L31 (-107.2972, 9.5792) -> (-107.2972, 12.2196)
  line L32 (-107.2972, 12.2196) -> (-107.2972, 14.86)
  line L33 (-107.2972, 14.86) -> (-106.3079, 14.5629)
  spline S181 degree 3 poles (-106.3079, 14.5629) (-105.7638, 14.3995) (-103.3761, 14.2824) (-101.0019, 14.3027) knots 0 0 0 0 1 1 1 1
  spline S182 degree 3 poles (-101.0019, 14.3027) (-96.2439, 14.3433) (-88.9622, 15.6813) (-83.9498, 17.4358) knots 0 0 0 0 1 1 1 1
  spline S183 degree 3 poles (-83.9498, 17.4358) (-80.6517, 18.5903) (-75.4519, 21.3453) (-71.8663, 23.838) knots 0 0 0 0 1 1 1 1
  spline S184 degree 3 poles (-71.8663, 23.838) (-69.2033, 25.6893) (-69.1019, 25.7253) (-66.3716, 25.7874) knots 0 0 0 0 1 1 1 1
  spline S185 degree 3 poles (-66.3716, 25.7874) (-64.3729, 25.8329) (-62.9027, 26.1116) (-61.1474, 26.7779) knots 0 0 0 0 1 1 1 1
  spline S186 degree 3 poles (-61.1474, 26.7779) (-58.9058, 27.6287) (-58.4913, 27.6768) (-56.1112, 27.3618) knots 0 0 0 0 1 1 1 1
  spline S187 degree 3 poles (-56.1112, 27.3618) (-53.4639, 27.0116) (-48.7211, 25.6297) (-46.8561, 24.6652) knots 0 0 0 0 1 1 1 1
  spline S188 degree 3 poles (-46.8561, 24.6652) (-46.2858, 24.3703) (-45.5279, 24.1266) (-45.1718, 24.1235) knots 0 0 0 0 1 1 1 1
  spline S189 degree 3 poles (-45.1718, 24.1235) (-44.8158, 24.1205) (-44.2816, 23.9645) (-43.9849, 23.7768) knots 0 0 0 0 1 1 1 1
  spline S190 degree 3 poles (-43.9849, 23.7768) (-43.1242, 23.2326) (-44.3044, 22.3149) (-46.1837, 22.0671) knots 0 0 0 0 1 1 1 1
  spline S191 degree 3 poles (-46.1837, 22.0671) (-47.0518, 21.9526) (-48.2629, 21.4794) (-48.8752, 21.0155) knots 0 0 0 0 1 1 1 1
  spline S192 degree 3 poles (-48.8752, 21.0155) (-50.1715, 20.0332) (-51.8278, 19.9308) (-53.386, 20.7366) knots 0 0 0 0 1 1 1 1
  spline S193 degree 3 poles (-53.386, 20.7366) (-54.937, 21.5386) (-55.9875, 21.4773) (-59.4346, 20.3836) knots 0 0 0 0 1 1 1 1
  spline S194 degree 3 poles (-59.4346, 20.3836) (-63.6558, 19.0442) (-65.2278, 18.8784) (-66.9965, 19.5861) knots 0 0 0 0 1 1 1 1
  spline S195 degree 3 poles (-66.9965, 19.5861) (-69.2699, 20.4957) (-69.97, 20.3294) (-72.6365, 18.2467) knots 0 0 0 0 1 1 1 1
  spline S196 degree 3 poles (-72.6365, 18.2467) (-76.2091, 15.4561) (-77.1108, 15.0663) (-79.681, 15.2012) knots 0 0 0 0 1 1 1 1
  spline S197 degree 3 poles (-79.681, 15.2012) (-82.797, 15.3647) (-82.9074, 14.5584) (-79.8143, 14.2271) knots 0 0 0 0 1 1 1 1
  spline S198 degree 3 poles (-79.8143, 14.2271) (-77.047, 13.9308) (-73.4302, 14.8564) (-71.1177, 16.4527) knots 0 0 0 0 1 1 1 1
  spline S199 degree 3 poles (-71.1177, 16.4527) (-69.8454, 17.331) (-69.3669, 17.4333) (-66.2881, 17.4848) knots 0 0 0 0 1 1 1 1
  spline S200 degree 3 poles (-66.2881, 17.4848) (-63.5423, 17.5308) (-62.385, 17.7298) (-60.3996, 18.4973) knots 0 0 0 0 1 1 1 1
  spline S201 degree 3 poles (-60.3996, 18.4973) (-56.9975, 19.8125) (-54.8172, 19.7811) (-52.857, 18.3886) knots 0 0 0 0 1 1 1 1
  spline S202 degree 3 poles (-52.857, 18.3886) (-51.6044, 17.4987) (-50.8927, 17.2897) (-48.5081, 17.1116) knots 0 0 0 0 1 1 1 1
  spline S203 degree 3 poles (-48.5081, 17.1116) (-46.9399, 16.9945) (-45.5234, 16.8162) (-45.3604, 16.7155) knots 0 0 0 0 1 1 1 1
  spline S204 degree 3 poles (-45.3604, 16.7155) (-45.1974, 16.6147) (-45.064, 15.8171) (-45.064, 14.943) knots 0 0 0 0 1 1 1 1
  spline S205 degree 3 poles (-45.064, 14.943) (-45.064, 13.6879) (-45.2342, 13.2451) (-45.8734, 12.8369) knots 0 0 0 0 1 1 1 1
  spline S206 degree 3 poles (-45.8734, 12.8369) (-46.5847, 12.3827) (-47.0971, 12.4022) (-50.1002, 12.9976) knots 0 0 0 0 1 1 1 1
  spline S207 degree 3 poles (-50.1002, 12.9976) (-55.2878, 14.0261) (-55.9849, 13.9621) (-57.1667, 12.3479) knots 0 0 0 0 1 1 1 1
  spline S208 degree 3 poles (-57.1667, 12.3479) (-57.71, 11.606) (-58.2675, 10.8625) (-58.4057, 10.6957) knots 0 0 0 0 1 1 1 1
  spline S209 degree 3 poles (-58.4057, 10.6957) (-58.5438, 10.5289) (-59.0764, 10.6673) (-59.5893, 11.0033) knots 0 0 0 0 1 1 1 1
  spline S210 degree 3 poles (-59.5893, 11.0033) (-60.3982, 11.5334) (-60.824, 11.5616) (-62.8048, 11.2167) knots 0 0 0 0 1 1 1 1
  spline S211 degree 3 poles (-62.8048, 11.2167) (-66.3038, 10.6074) (-68.6108, 10.7106) (-69.9666, 11.5372) knots 0 0 0 0 1 1 1 1
  spline S212 degree 3 poles (-69.9666, 11.5372) (-70.6821, 11.9734) (-71.7798, 12.2556) (-72.7632, 12.2561) knots 0 0 0 0 1 1 1 1
  spline S213 degree 3 poles (-72.7632, 12.2561) (-73.6535, 12.2566) (-76.1296, 12.4463) (-78.2657, 12.6777) knots 0 0 0 0 1 1 1 1
  spline S214 degree 3 poles (-78.2657, 12.6777) (-82.7419, 13.1625) (-82.4963, 13.2752) (-84.2766, 9.9198) knots 0 0 0 0 1 1 1 1
  spline S215 degree 3 poles (-84.2766, 9.9198) (-86.6943, 5.363) (-89.0079, 4.2599) (-93.0879, 5.7188) knots 0 0 0 0 1 1 1 1
  spline S216 degree 3 poles (-93.0879, 5.7188) (-95.0605, 6.4242) (-101.4381, 7.3304) (-102.977, 7.124) knots 0 0 0 0 1 1 1 1
  spline S217 degree 3 poles (-102.977, 7.124) (-104.6778, 6.8959) (-109.5175, 3.8363) (-111.5946, 1.6762) knots 0 0 0 0 1 1 1 1
  spline S218 degree 3 poles (-111.5946, 1.6762) (-112.6737, 0.5539) (-113.7723, -0.0018) (-113.7723, 0.5747) knots 0 0 0 0 1 1 1 1
  spline S219 degree 3 poles (-103.6099, 16.7551) (-104.4176, 17.3338) (-104.7005, 19.0207) (-104.2061, 20.3092) knots 0 0 0 0 1 1 1 1
  spline S220 degree 3 poles (-104.2061, 20.3092) (-103.9516, 20.9725) (-99.2648, 22.8371) (-95.8712, 23.6252) knots 0 0 0 0 1 1 1 1
  spline S221 degree 3 poles (-95.8712, 23.6252) (-94.3002, 23.99) (-92.7889, 24.106) (-91.575, 23.9548) knots 0 0 0 0 1 1 1 1
  spline S222 degree 3 poles (-91.575, 23.9548) (-90.1035, 23.7715) (-89.3445, 23.8798) (-88.0319, 24.4604) knots 0 0 0 0 1 1 1 1
  spline S223 degree 3 poles (-88.0319, 24.4604) (-85.9604, 25.3768) (-83.1877, 27.3824) (-80.9584, 29.5772) knots 0 0 0 0 1 1 1 1
  spline S224 degree 3 poles (-80.9584, 29.5772) (-79.1578, 31.3498) (-76.7938, 32.4028) (-74.6147, 32.4028) knots 0 0 0 0 1 1 1 1
  spline S225 degree 3 poles (-74.6147, 32.4028) (-73.9229, 32.4028) (-72.1577, 31.9889) (-70.6919, 31.483) knots 0 0 0 0 1 1 1 1
  spline S226 degree 3 poles (-70.6919, 31.483) (-67.1326, 30.2545) (-64.8526, 30.0029) (-63.5386, 30.6936) knots 0 0 0 0 1 1 1 1
  spline S227 degree 3 poles (-63.5386, 30.6936) (-62.9734, 30.9908) (-61.948, 31.5271) (-61.2601, 31.8855) knots 0 0 0 0 1 1 1 1
  spline S228 degree 3 poles (-61.2601, 31.8855) (-59.5312, 32.7861) (-56.6056, 32.9849) (-55.2852, 32.2915) knots 0 0 0 0 1 1 1 1
  spline S229 degree 3 poles (-55.2852, 32.2915) (-53.7323, 31.4759) (-51.0459, 28.5932) (-51.3621, 28.0816) knots 0 0 0 0 1 1 1 1
  spline S230 degree 3 poles (-51.3621, 28.0816) (-51.5552, 27.7691) (-52.385, 27.7219) (-54.3718, 27.9102) knots 0 0 0 0 1 1 1 1
  spline S231 degree 3 poles (-54.3718, 27.9102) (-58.2574, 28.2785) (-60.2188, 28.184) (-62.1252, 27.5368) knots 0 0 0 0 1 1 1 1
  spline S232 degree 3 poles (-62.1252, 27.5368) (-63.3075, 27.1354) (-64.3899, 27.0413) (-65.8829, 27.2102) knots 0 0 0 0 1 1 1 1
  spline S233 degree 3 poles (-65.8829, 27.2102) (-68.3593, 27.4904) (-69.6868, 27.0014) (-74.0747, 24.1928) knots 0 0 0 0 1 1 1 1
  spline S234 degree 3 poles (-74.0747, 24.1928) (-77.1252, 22.2403) (-78.7166, 21.5378) (-84.8141, 19.4519) knots 0 0 0 0 1 1 1 1
  spline S235 degree 3 poles (-84.8141, 19.4519) (-89.2878, 17.9215) (-91.2646, 17.478) (-96.1456, 16.9097) knots 0 0 0 0 1 1 1 1
  spline S236 degree 3 poles (-96.1456, 16.9097) (-102.7132, 16.145) (-102.7571, 16.1441) (-103.6099, 16.7551) knots 0 0 0 0 1 1 1 1
  spline S237 degree 3 poles (-94.5268, 27.5299) (-97.0161, 28.0518) (-97.9442, 28.4015) (-97.9442, 28.8175) knots 0 0 0 0 1 1 1 1
  spline S238 degree 3 poles (-97.9442, 28.8175) (-97.9442, 29.1394) (-90.5724, 33.1871) (-81.6804, 37.7475) knots 0 0 0 0 1 1 1 1
  line L34 (-81.6804, 37.7475) -> (-76.0286, 40.6461)
  line L35 (-76.0286, 40.6461) -> (-74.1508, 40.0885)
  spline S239 degree 3 poles (-74.1508, 40.0885) (-72.862, 39.7057) (-71.6679, 39.6064) (-70.3436, 39.7719) knots 0 0 0 0 1 1 1 1
  spline S240 degree 3 poles (-70.3436, 39.7719) (-68.7561, 39.9702) (-68.15, 39.8753) (-66.9242, 39.2363) knots 0 0 0 0 1 1 1 1
  spline S241 degree 3 poles (-66.9242, 39.2363) (-65.7641, 38.6317) (-64.9515, 38.4861) (-63.2531, 38.5789) knots 0 0 0 0 1 1 1 1
  spline S242 degree 3 poles (-63.2531, 38.5789) (-61.2423, 38.6888) (-61.0633, 38.6368) (-60.9603, 37.9136) knots 0 0 0 0 1 1 1 1
  spline S243 degree 3 poles (-60.9603, 37.9136) (-60.8733, 37.3025) (-61.4321, 36.69) (-63.4894, 35.1415) knots 0 0 0 0 1 1 1 1
  spline S244 degree 3 poles (-63.4894, 35.1415) (-67.3963, 32.201) (-67.7897, 32.0846) (-71.9618, 32.6349) knots 0 0 0 0 1 1 1 1
  spline S245 degree 3 poles (-71.9618, 32.6349) (-79.0007, 33.5632) (-79.9806, 33.3515) (-85.5155, 29.7064) knots 0 0 0 0 1 1 1 1
  spline S246 degree 3 poles (-85.5155, 29.7064) (-89.8059, 26.881) (-90.5614, 26.6985) (-94.5268, 27.5299) knots 0 0 0 0 1 1 1 1
  spline S247 degree 3 poles (-87.2423, 37.4678) (-88.2155, 38.0347) (-87.9884, 38.7952) (-86.7659, 39.0637) knots 0 0 0 0 1 1 1 1
  spline S248 degree 3 poles (-86.7659, 39.0637) (-86.1576, 39.1973) (-85.1174, 39.783) (-84.4542, 40.3653) knots 0 0 0 0 1 1 1 1
  spline S249 degree 3 poles (-84.4542, 40.3653) (-83.5753, 41.137) (-82.2902, 41.6678) (-79.7145, 42.3232) knots 0 0 0 0 1 1 1 1
  spline S250 degree 3 poles (-79.7145, 42.3232) (-75.7287, 43.3373) (-73.7334, 43.3574) (-73.5492, 42.3853) knots 0 0 0 0 1 1 1 1
  spline S251 degree 3 poles (-73.5492, 42.3853) (-73.4477, 41.8499) (-73.7161, 41.7554) (-75.3448, 41.7534) knots 0 0 0 0 1 1 1 1
  spline S252 degree 3 poles (-75.3448, 41.7534) (-76.6649, 41.7518) (-77.5951, 41.5258) (-78.339, 41.026) knots 0 0 0 0 1 1 1 1
  spline S253 degree 3 poles (-78.339, 41.026) (-79.4681, 40.2674) (-86.007, 37.0713) (-86.3911, 37.0902) knots 0 0 0 0 1 1 1 1
  spline S254 degree 3 poles (-86.3911, 37.0902) (-86.513, 37.0963) (-86.896, 37.2662) (-87.2423, 37.4678) knots 0 0 0 0 1 1 1 1
  line L36 (-75.5, 47.5) -> (-79.5, 47.5)
  line L37 (-79.5, 47.5) -> (-79.5, 49.5)
  line L38 (-79.5, 49.5) -> (-75.5, 49.5)
  line L39 (-75.5, 49.5) -> (-75.5, 47.5)
  line L40 (0, 0) -> (-2, 0)
  line L41 (-2, 0) -> (-2, 4)
  line L42 (-2, 4) -> (0, 4)
  line L43 (0, 4) -> (0, 0)
  line L44 (0, 0) -> (-2, 4) construction
  line L45 (-2, 0) -> (0, 4) construction
  line L46 (-155, 4) -> (-153, 4)
  line L47 (-153, 4) -> (-153, 0)
  line L48 (-153, 0) -> (-155, 0)
  line L49 (-155, 0) -> (-155, 4)
  line L50 (-155, 4) -> (-153, 0) construction
  line L51 (-153, 4) -> (-155, 0) construction
  circle A0 centre (-4.1421, 45.3579) radius 1
  circle A1 centre (-4.1421, 45.3579) radius 1
  circle A2 centre (-4.1421, -41.3579) radius 1
  circle A3 centre (-150.8579, -41.3579) radius 1
  circle A4 centre (-150.8579, 45.3579) radius 1
  point P0 (0, 49.5)
  point P1 (-155, -45.5)
  point P2 (-77.5, 2)
  point P3 (-77.5, 2)
  point P4 (2, 51.5)
  point P5 (-77.5, 49.5)
  point P6 (-77.5, 49.5)
  point P7 (-77.5, 49.5)
  point P8 (-1, 2)
  point P9 (0, 2)
  point P10 (-155, 2)
  point P11 (0, 2)
  point P12 (-154, 2)
  point P13 (-155, 2)
  point P14 (-14.1421, 49.5)
  point P15 (0, 49.5)
  point P16 (0, -31.3579)
  point P17 (-4.1421, -41.3579)
  point P18 (-155, -31.3579)
  point P19 (-150.8579, -41.3579)
  point P20 (-140.8579, 49.5)
  point P21 (-150.8579, 45.3579)
  dimension "d74" = 4
  dimension "d75" = 2
  dimension "d78" = 2
  dimension "d79" = 4
  dimension "d80" = 2
  dimension "d81" = 4
  dimension "d117" = 14.1421
  dimension "d118" = 2
  dimension "d120" = 22.5
  dimension "d121" = 2
  dimension "d123" = 14.1421
  dimension "d124" = 45
  dimension "d125" = 45
  dimension "d126" = 22.5
  dimension "d127" = 2
  dimension "d128" = 14.1421
  dimension "d129" = 45
  dimension "d130" = 22.5
  dimension "d131" = 2
  dimension "d132" = 14.1421
  dimension "d133" = 22.5
  dimension "d134" = 45
  dimension "d135" = 2
  constraint horizontal L0
  constraint vertical L1
  constraint horizontal L2
  constraint vertical L3
  constraint coincident P15 P0
  constraint coincident P1 L1.end
  constraint coincident L4 P3
  constraint coincident L5 P3
  constraint horizontal L6
  constraint perpendicular L6 L7
  constraint parallel L6 L8
  constraint parallel L7 L9
  constraint coincident L10 P3
  constraint coincident L11 P3
  constraint coincident P3 P2
  constraint coincident P4 L6.start
  constraint coincident L7 L12.end
  constraint perpendicular L7 L12
  constraint coincident L9 L13.end
  constraint perpendicular L9 L13
  constraint horizontal L36
  constraint vertical L37
  constraint horizontal L38
  constraint vertical L39
  constraint midpoint L38 P7
  constraint midpoint L0 P7
  constraint coincident P7 P6
  constraint horizontal L40
  constraint perpendicular L40 L41
  constraint parallel L40 L42
  constraint parallel L41 L43
  constraint coincident L44 P8
  constraint coincident L45 P8
  constraint midpoint L43 P11
  constraint midpoint L1 P13
  constraint midpoint L3 P11
  constraint coincident P11 P9
  constraint horizontal L46
  constraint perpendicular L46 L47
  constraint parallel L46 L48
  constraint parallel L47 L49
  constraint coincident L50 P12
  constraint coincident L51 P12
  constraint midpoint L49 P13
  constraint coincident P13 P10
  constraint coincident L0 P14
  constraint coincident L3 P16
  constraint coincident P17 A2.centre
  constraint coincident L1 P18
  constraint coincident P19 A3.centre
  constraint coincident L0 P20
  constraint coincident P21 A4.centre
  measures "d74" distance of L36.start L36.end
  measures "d75" distance of L36.start L38.end
  measures "d78" distance of L41.end L42.end
  measures "d79" distance of L40.end L41.end
  measures "d80" distance of L47.end L48.end
  measures "d81" distance of L46.end L47.end
  measures "d117" distance of P15 P14
  measures "d118" diameter of A0
  measures "d120" angle of P15 P14 A0.centre
  measures "d121" diameter of A1
  measures "d123" distance of L2.end P16
  measures "d124" angle of P14 A0.centre P15
  measures "d125" angle of L2.end P16 P17
  measures "d126" angle of L2.end P16 P17
  measures "d127" diameter of A2
  measures "d128" distance of P1 P18
  measures "d129" angle of P1 P18 P19
  measures "d130" angle of P1 P18 P19
  measures "d131" diameter of A3
  measures "d132" distance of L0.end P20
  measures "d133" angle of L0.end P20 P21
  measures "d134" angle of L0.end P20 P21